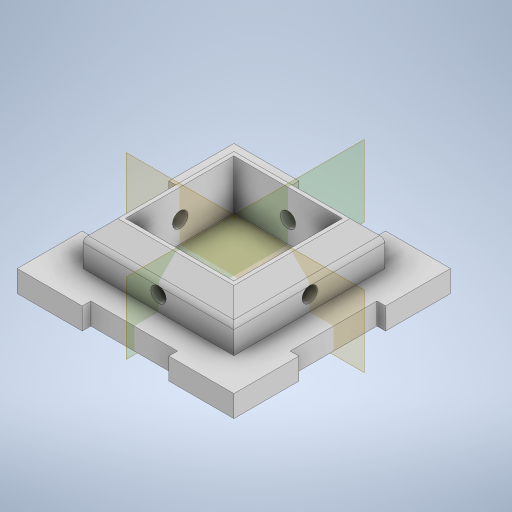
# Autodesk Inventor part: Pokrywka
Saved by Autodesk Inventor 2024 (Build 280153000, 153)
## iProperties
Created: 2023-10-17
Part Number: Pokrywka
Material: Generic
Document SubType Name: Modeling
Designer: Piter
Density: 1 g/cm^3
Appearance: Default
Author: Piter
Autodesk Inventor part; units mm, degrees
ref_plane "YZ Plane" through (0, 0, 0) normal (1, 0, 0) x (0, 1, 0)
ref_plane "XZ Plane" through (0, 0, 0) normal (0, 1, 0) x (-1, 0, 0)
ref_plane "XY Plane" through (0, 0, 0) normal (0, 0, 1) x (1, 0, 0)
sketch "Sketch1" plane through (0, 0, 0) normal (0, 1, 0) x (-1, 0, 0)
  line L0 (-25, 25) -> (25, 25)
  line L1 (25, 25) -> (25, -25)
  line L2 (25, -25) -> (-25, -25)
  line L3 (-25, -25) -> (-25, 25)
  line L4 (-25, 25) -> (25, -25) construction
  line L5 (25, 25) -> (-25, -25) construction
  line L6 (-17.4, 17.4) -> (17.4, 17.4)
  line L7 (17.4, 17.4) -> (17.4, -17.4)
  line L8 (17.4, -17.4) -> (-17.4, -17.4)
  line L9 (-17.4, -17.4) -> (-17.4, 17.4)
  line L10 (-17.4, 17.4) -> (17.4, -17.4) construction
  line L11 (17.4, 17.4) -> (-17.4, -17.4) construction
  point P0 (0, 0)
  dimension "d0" = 50
  dimension "d1" = 50
  dimension "d2" = 34.8
  dimension "d3" = 34.8
  constraints: 24 end point, 4 midpoint, 4 parallel, 2 horizontal, 2 perpendicular
  measures "d0" distance of L1.end L2.end
  measures "d1" distance of L0.end L1.end
  measures "d2" distance of L7.end L8.end
  measures "d3" distance of L6.end L7.end
extrude "Extrusion1" add sketch "Sketch1" along normal blind 5
extrude "Extrusion2" add sketch "Sketch1" along normal blind 15 contours L6 L7 L8 L9
sketch "Sketch3" plane through (0, 15, 0) normal (0, 1, 0) x (1, 0, 0)
  point P0 (0, 0)
ref_plane "Work Plane6" through (0, 5, 17.4) normal (-1, 0, 0) x (0, 0, 1)
ref_plane "Work Plane7" through (-17.4, 5, 0) normal (0, 0, 1) x (1, 0, 0)
sketch "Sketch6" plane through (0, 0, 0) normal (0, -1, 0) x (1, 0, 0)
  line L0 (-25, 25) -> (25, 25) projected
  line L1 (-5, -25) -> (5, -25)
  line L2 (5, -25) -> (5, 25)
  line L3 (5, 25) -> (-5, 25)
  line L4 (-5, 25) -> (-5, -25)
  line L5 (-5, -25) -> (5, 25) construction
  line L6 (5, -25) -> (-5, 25) construction
  line L7 (25, 25) -> (25, -25) projected
  line L8 (-25, -5) -> (25, -5)
  line L9 (25, -5) -> (25, 5)
  line L10 (25, 5) -> (-25, 5)
  line L11 (-25, 5) -> (-25, -5)
  line L12 (-25, -5) -> (25, 5) construction
  line L13 (25, -5) -> (-25, 5) construction
  point P0 (0, 0)
  point P1 (-5, -5)
  point P2 (5, -5)
  point P3 (5, 5)
  point P4 (-5, 5)
  dimension "d14" = 10
  constraints: 24 end point, 4 midpoint, 4 parallel, 2 horizontal, 2 perpendicular, 2 point on line
  measures "d14" distance of L3.end L2.end
extrude "Extrusion5" add sketch "Sketch6" along normal blind 2 contours L0 L2 L10 L4 | L10 L2 L8 L4 | L4 L8 L11 L10 | L10 L7 L8 L2 | L8 L2 L1 L4
sketch "Sketch7" plane through (-25, 0, 25) normal (-1, 0, 0) x (0, 0, 1)
  line L0 (-20, -2) -> (-30, -2) projected
  line L1 (-7.6, 5) -> (-42.4, 5) projected
  line L2 (-20, -2) -> (-30, -2)
  line L3 (-30, -2) -> (-30, 5)
  line L4 (-30, 5) -> (-20, 5)
  line L5 (-20, 5) -> (-20, -2)
  point P0 (-25, 0)
  dimension "d17" = 10
  constraints: 8 end point, 2 parallel, 1 horizontal, 1 perpendicular, 1 point on line
  measures "d17" distance of L3.end L4.end
extrude "Extrusion6" add sketch "Sketch7" along normal blind 2
mirror "Mirror4" about plane through (0, 5, 17.4) normal (-1, 0, 0) of "Extrusion6"
sketch "Sketch8" plane through (25, 5, -25) normal (0, 0, -1) x (-1, 0, 0)
  line L0 (30, -7) -> (20, -7) projected
  line L1 (0, 0) -> (50, 0) projected
  line L2 (20, -7) -> (30, -7)
  line L3 (30, -7) -> (30, 0)
  line L4 (30, 0) -> (20, 0)
  line L5 (20, 0) -> (20, -7)
  point P0 (25, -5)
  dimension "d20" = 10
  constraints: 8 end point, 2 parallel, 1 horizontal, 1 perpendicular, 1 point on line
  measures "d20" distance of L4.end L3.end
extrude "Extrusion7" add sketch "Sketch8" along normal blind 2
mirror "Mirror5" about plane through (-17.4, 5, 0) normal (0, 0, 1) of "Extrusion7"
sketch "Sketch9" plane through (0, 0, 0) normal (0, -1, 0) x (1, 0, 0)
  line L0 (-27, 27) -> (27, 27)
  line L1 (27, 27) -> (27, -27)
  line L2 (27, -27) -> (-27, -27)
  line L3 (-27, -27) -> (-27, 27)
  line L4 (-27, 27) -> (27, -27) construction
  line L5 (27, 27) -> (-27, -27) construction
  point P0 (0, 0)
  dimension "d24" = 54
  dimension "d25" = 54
  constraints: 12 end point, 2 midpoint, 2 parallel, 1 horizontal, 1 perpendicular
  measures "d24" distance of L1.end L2.end
  measures "d25" distance of L0.end L1.end
extrude "Extrusion8" cut sketch "Sketch9" along normal blind 6.75
sketch "Sketch10" plane through (0, 15, 0) normal (0, 1, 0) x (1, 0, 0)
  line L0 (12.5, -12.5) -> (-12.5, -12.5)
  line L1 (-12.5, -12.5) -> (-12.5, 12.5)
  line L2 (-12.5, 12.5) -> (12.5, 12.5)
  line L3 (12.5, 12.5) -> (12.5, -12.5)
  line L4 (12.5, -12.5) -> (-12.5, 12.5) construction
  line L5 (-12.5, -12.5) -> (12.5, 12.5) construction
  point P0 (0, 0)
  dimension "d28" = 25
  dimension "d29" = 25
  constraints: 12 end point, 2 midpoint, 2 parallel, 1 horizontal, 1 perpendicular
  measures "d28" distance of L1.end L2.end
  measures "d29" distance of L0.end L1.end
extrude "Extrusion9" cut sketch "Sketch10" against normal blind 11.45
sketch "Sketch11" plane through (-17.4, 5, 17.4) normal (-1, 0, 0) x (0, 0, 1)
  line L0 (-17.5, 0.0162) -> (-17.5, 3.5)
  circle A0 centre (-17.5, 3.5) radius 1.75
  line L1 (0, 0) -> (-34.8, 0) projected
  line L2 (-17.4, 0) -> (-18.8366, 0)
  point P0 (-17.4, -5)
  dimension "d34" = 3.5
  dimension "d57" = 3.5
  constraints: 4 end point, 1 centre point, 1 coincident, 1 midpoint, 1 point on line, 1 vertical
  measures "d34" diameter of A0
  measures "d57" distance from line of L1 L0.end
extrude "Extrusion10" cut sketch "Sketch11" against normal through all
sketch "Sketch14" plane through (27, 0, -5) normal (1, 0, 0) x (0, 0, -1)
  line L0 (12.4, 5) -> (-22.4, 5) projected
  line L1 (-15, 0) -> (5, 0)
  line L2 (5, 0) -> (5, 5)
  line L3 (5, 5) -> (-15, 5)
  line L4 (-15, 5) -> (-15, 0)
  line L5 (-15, 0) -> (5, 5) construction
  line L6 (5, 0) -> (-15, 5) construction
  point P0 (-5, 0)
  point P1 (-5, 2.5)
  dimension "d43" = 20
  constraints: 12 end point, 2 midpoint, 2 parallel, 1 horizontal, 1 perpendicular, 1 point on line
  measures "d43" distance of L3.end L2.end
extrude "Extrusion13" cut sketch "Sketch14" against normal blind 4
pattern_circular "Circular Pattern1" count 4 over 360 about axis through (0, -10, 0) along (0, 1, 0) of "Extrusion13"
sketch "Sketch15" plane through (17.4, 5, -17.4) normal (0, 0, -1) x (-1, 0, 0)
  line L0 (27.4, 0) -> (7.4, 0) projected
  line L1 (17.4, 0) -> (17.4, 3.5)
  circle A0 centre (17.4, 3.5) radius 1.75
  point P0 (17.4, -5)
  dimension "d49" = 3.5
  dimension "d50" = 3.5
  constraints: 2 end point, 1 centre point, 1 coincident, 1 midpoint, 1 vertical
  measures "d49" distance of L1.start L1.end
  measures "d50" diameter of A0
extrude "Extrusion14" cut sketch "Sketch15" against normal through all
chamfer "Chamfer1" distance 4 distance2 4 4 edges at (0, 15, -17.4) (-17.4, 15, 0) (0, 15, 17.4) (17.4, 15, 0) measured on face at (0, 15, -16.9) measured on face at (16.9, 15, 0) measured on face at (0, 15, 16.9) measured on face at (-16.9, 15, 0)
fillet "Fillet1" radius 2 4 edges at (0, 11, -17.4) (-17.4, 11, 0) (0, 11, 17.4) (17.4, 11, 0)
body "Solid1"
